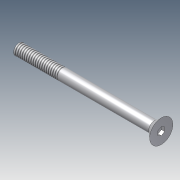
# Autodesk Inventor part: HW-00073
Saved by Autodesk Inventor 2012 (Build 160160000, 160)
## iProperties
Created: 2008-05-28
Part Number: HW-00073
Document SubType Name: Modeling
Designer: mcyr
Density: 1 g/cm^3
Mass: 1.98402 g
Surface Area: 14.2837 cm^2
Volume: 1.98402 cm^3
Description: FHCS 1/4-20 x 3-1/4"
Material: Default
Title: FHCS 1/4-20 x 3-1/4"
Author: mcyr
Autodesk Inventor part; units mm, degrees
ref_plane "YZ Plane" through (0, 0, 0) normal (1, 0, 0) x (0, 1, 0)
ref_plane "XZ Plane" through (0, 0, 0) normal (0, 1, 0) x (-1, 0, 0)
ref_plane "XY Plane" through (0, 0, 0) normal (0, 0, 1) x (1, 0, 0)
sketch "Sketch1" plane through (0, 0, 0) normal (0, 0, 1) x (1, 0, 0)
  line L0 (-12.5919, 2.2112) -> (69.9581, 2.2112)
  line L1 (69.9581, 2.2112) -> (69.9581, 8.9549)
  line L2 (69.9581, 8.9549) -> (65.8687, 5.3862)
  line L3 (65.8687, 5.3862) -> (-12.5919, 5.3862)
  line L4 (-12.5919, 5.3862) -> (-12.5919, 2.2112)
  dimension "d0" = 3.175
  dimension "d2" = 4.0894
  dimension "d3" = 6.7437
  dimension "d19" = 82.55
  constraints: 10 end point, 2 parallel, 1 horizontal, 1 perpendicular
  measures "d0" distance of L3.end L0.start
  measures "d2" horizontal distance of L1.end L2.end
  measures "d3" distance of L0.end L1.end
  measures "d19" distance of L0.start L0.end
revolve "Revolution1" add sketch "Sketch1" angle 360 about axis through (-12.5919, 2.2112, 0) along (1, 0, 0)
thread "Thread1" size "1/4-20 UNC" class "2A" standard "ANSI Unified Screw Threads" length 25.4
sketch "Sketch2" plane through (69.9581, 2.2112, 0) normal (1, 0, 0) x (0, 0, -1)
  circle A0 centre (0, 0) radius 6.7437 projected
  line L0 (0, -2.2914) -> (-1.9844, -1.1457)
  line L1 (-1.9844, -1.1457) -> (-1.9844, 1.1457)
  line L2 (-1.9844, 1.1457) -> (0, 2.2914)
  line L3 (0, 2.2914) -> (1.9844, 1.1457)
  line L4 (1.9844, 1.1457) -> (1.9844, -1.1457)
  line L5 (1.9844, -1.1457) -> (0, -2.2914)
  dimension "d16" = 3.9688
  constraints: 12 end point, 1 coincident, 13 other
  measures "d16" distance between parallel lines of L4 L1
extrude "Extrusion1" cut sketch "Sketch2" against normal blind 1.905 contours L0 L1 L2 L3 L4 L5
body "Solid1"
